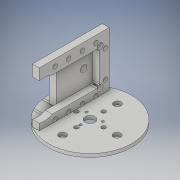
# Autodesk Inventor part: база захвата
Saved by Autodesk Inventor 2019 (Build 230136000, 136)
## iProperties
Created: 2019-08-15
Part Number: база захвата
Material: Типовые
Document SubType Name: Modeling
Designer: Петров Иван
Density: 1 g/cm^3
Appearance: По умолчанию
Author: Петров Иван
Autodesk Inventor part; units mm, degrees
ref_plane "YZ Plane" through (0, 0, 0) normal (1, 0, 0) x (0, 1, 0)
ref_plane "XZ Plane" through (0, 0, 0) normal (0, 1, 0) x (-1, 0, 0)
ref_plane "XY Plane" through (0, 0, 0) normal (0, 0, 1) x (1, 0, 0)
sketch "Эскиз1" plane through (0, 0, 0) normal (0, 1, 0) x (-1, 0, 0)
  circle A0 centre (15.9998, -0.0856) radius 2.1
  circle A1 centre (-15.9998, 0.0856) radius 2.1
  circle A2 centre (0.0856, 15.9998) radius 2.1
  circle A3 centre (-0.0856, -15.9998) radius 2.1
  circle A4 centre (0, 0) radius 2.9
  circle A5 centre (8, 0) radius 1.25
  circle A6 centre (0, 8) radius 1.25
  circle A7 centre (-8, 0) radius 1.25
  circle A8 centre (4.7631, -2.75) radius 0.75
  circle A9 centre (-4.7631, -2.75) radius 0.75
  circle A10 centre (0, 5.5) radius 0.75
  circle A11 centre (0, -8) radius 1.25
  circle A12 centre (0, 0) radius 24.5
  constraints: 13 centre point
extrude "Выдавливание1" add sketch "Эскиз1" along normal blind 2
sketch "Эскиз2" plane through (0, 2, 0) normal (0, 1, 0) x (1, 0, 0)
  line L0 (-13.1408, -20.6607) -> (-9.1408, -20.6607)
  line L1 (-9.1408, -20.6607) -> (-9.1408, 20.3393)
  line L2 (-9.1408, 20.3393) -> (-13.1408, 20.3393)
  line L3 (-13.1408, 20.3393) -> (-13.1408, -20.6607)
  circle A0 centre (0, 0) radius 24.5 projected
  dimension "d2" = 4
  dimension "d3" = 41
  dimension "d4" = 20.3393
  constraints: 8 end point, 2 parallel, 1 horizontal, 1 perpendicular
  measures "d2" distance of L2.end L1.end
  measures "d3" distance of L1.end L0.end
  measures "d4" distance from line of A0.centre L2
extrude "Выдавливание2" add sketch "Эскиз2" along normal blind 32 contours L3 L2 L1 L0
sketch "Эскиз3" plane through (-9.1408, 2, 20.6607) normal (1, 0, 0) x (0, 0, -1)
  line L0 (20.5612, 2.0176) -> (20.5612, -0.2824)
  line L1 (20.5612, 2.0176) -> (21.9612, 2.0176)
  line L2 (21.9612, -0.2824) -> (21.9612, 2.0176)
  line L3 (28.5612, -0.2824) -> (21.9612, -0.2824)
  line L4 (28.5612, 2.0176) -> (28.5612, -0.2824)
  circle A0 centre (2.7612, 14.6176) radius 9.15
  circle A1 centre (2.7612, 14.6176) radius 1.5
  circle A2 centre (38.7612, 22.6176) radius 1.3
  circle A3 centre (25.2612, 28.1176) radius 1.3
  circle A4 centre (33.2612, 28.1176) radius 1.3
  circle A5 centre (17.2612, 28.1176) radius 1.3
  circle A6 centre (9.2612, 28.1176) radius 1.3
  circle A7 centre (38.7612, 6.6176) radius 1.3
  circle A8 centre (25.2612, 1.1176) radius 1.3
  circle A9 centre (33.2612, 1.1176) radius 1.3
  circle A10 centre (17.2612, 1.1176) radius 1.3
  circle A11 centre (9.2612, 1.1176) radius 1.3
  line L5 (-8.2587, 14.5176) -> (-7.7184, 14.5176)
  line L6 (-8.2587, 7.6176) -> (-8.2587, 14.5176)
  arc A12 (-8.2587, 7.6176) -> (-8.2075, 6.8676) centre (-2.7388, 7.6176) ccw
  line L7 (-5.7388, 6.8676) -> (-8.2075, 6.8676)
  arc A13 (-3.9888, 5.1176) -> (-5.7388, 6.8676) centre (-5.7388, 5.1176) ccw
  line L8 (-3.9888, 4.6176) -> (-3.9888, 5.1176)
  line L9 (33.5674, 4.6176) -> (-3.9888, 4.6176)
  arc A14 (33.5674, 4.6176) -> (34.2556, 5.0098) centre (33.5674, 5.4176) ccw
  arc A15 (34.2556, 5.0098) -> (34.869, 5.6231) centre (35.7612, 4.1176) ccw
  arc A16 (34.869, 5.6231) -> (35.2612, 6.3114) centre (34.4612, 6.3114) ccw
  line L10 (35.2612, 22.9239) -> (35.2612, 6.3114)
  arc A17 (35.2612, 22.9239) -> (34.869, 23.6121) centre (34.4612, 22.9239) ccw
  arc A18 (34.2556, 24.2255) -> (34.869, 23.6121) centre (35.7612, 25.1176) ccw
  arc A19 (34.869, 23.6121) -> (34.2556, 24.2255) centre (35.7612, 25.1176) ccw
  line L11 (-3.9888, 3.2947) -> (-3.9888, 4.6176)
  arc A20 (-3.9888, 3.2947) -> (-2.7388, 3.1176) centre (-2.7377, 7.6254) ccw
  line L12 (-2.7388, 3.1176) -> (4.7612, 3.1176)
  line L13 (4.7612, 2.0176) -> (4.7612, 3.1176)
  line L14 (5.9612, 2.0176) -> (4.7612, 2.0176)
  line L15 (5.9612, -0.2824) -> (5.9612, 2.0176)
  line L16 (12.5612, -0.2824) -> (5.9612, -0.2824)
  line L17 (12.5612, 2.0176) -> (12.5612, -0.2824)
  line L18 (13.9612, 2.0176) -> (12.5612, 2.0176)
  line L19 (13.9612, -0.2824) -> (13.9612, 2.0176)
  line L20 (20.5612, -0.2824) -> (13.9612, -0.2824)
  line L21 (20.5612, 2.0176) -> (20.5612, -0.2824)
  line L22 (21.9612, 2.0176) -> (20.5612, 2.0176)
  line L23 (21.9612, -0.2824) -> (21.9612, 2.0176)
  line L24 (28.5612, -0.2824) -> (21.9612, -0.2824)
  line L25 (28.5612, 2.0176) -> (28.5612, -0.2824)
  line L26 (29.9612, 2.0176) -> (28.5612, 2.0176)
  line L27 (29.9612, -0.2824) -> (29.9612, 2.0176)
  line L28 (36.5612, -0.2824) -> (29.9612, -0.2824)
  line L29 (36.5612, 2.0176) -> (36.5612, -0.2824)
  line L30 (37.781, 2.0176) -> (36.5612, 2.0176)
  arc A21 (37.781, 2.0176) -> (37.8612, 2.0978) centre (36.7612, 3.1176) ccw
  line L31 (37.8612, 3.3176) -> (37.8612, 2.0978)
  line L32 (40.1612, 3.3176) -> (37.8612, 3.3176)
  line L33 (40.1612, 9.9176) -> (40.1612, 3.3176)
  line L34 (37.8612, 9.9176) -> (40.1612, 9.9176)
  line L35 (37.8612, 19.3176) -> (37.8612, 9.9176)
  line L36 (40.1612, 19.3176) -> (37.8612, 19.3176)
  line L37 (40.1612, 25.9176) -> (40.1612, 19.3176)
  line L38 (37.8612, 25.9176) -> (40.1612, 25.9176)
  line L39 (37.8612, 27.1374) -> (37.8612, 25.9176)
  arc A22 (37.8612, 27.1374) -> (37.781, 27.2176) centre (36.7612, 26.1176) ccw
  line L40 (36.5612, 27.2176) -> (37.781, 27.2176)
  line L41 (36.5612, 29.5176) -> (36.5612, 27.2176)
  line L42 (29.9612, 29.5176) -> (36.5612, 29.5176)
  line L43 (29.9612, 27.2176) -> (29.9612, 29.5176)
  line L44 (28.5612, 27.2176) -> (29.9612, 27.2176)
  line L45 (28.5612, 29.5176) -> (28.5612, 27.2176)
  line L46 (21.9612, 29.5176) -> (28.5612, 29.5176)
  line L47 (21.9612, 27.2176) -> (21.9612, 29.5176)
  line L48 (20.5612, 27.2176) -> (21.9612, 27.2176)
  line L49 (20.5612, 29.5176) -> (20.5612, 27.2176)
  line L50 (13.9612, 29.5176) -> (20.5612, 29.5176)
  line L51 (13.9612, 27.2176) -> (13.9612, 29.5176)
  line L52 (12.5612, 27.2176) -> (13.9612, 27.2176)
  line L53 (12.5612, 29.5176) -> (12.5612, 27.2176)
  line L54 (5.9612, 29.5176) -> (12.5612, 29.5176)
  line L55 (5.9612, 27.2176) -> (5.9612, 29.5176)
  line L56 (4.7612, 27.2176) -> (5.9612, 27.2176)
  line L57 (4.7612, 26.1176) -> (4.7612, 27.2176)
  line L58 (-2.7388, 26.1176) -> (4.7612, 26.1176)
  arc A23 (-2.7388, 26.1176) -> (-3.9888, 25.9405) centre (-2.7377, 21.6098) ccw
  line L59 (-3.9888, 24.6176) -> (-3.9888, 25.9405)
  line L60 (-3.9888, 24.1176) -> (-3.9888, 24.6176)
  arc A24 (-5.7388, 22.3676) -> (-3.9888, 24.1176) centre (-5.7388, 24.1176) ccw
  line L61 (-8.2075, 22.3676) -> (-5.7388, 22.3676)
  arc A25 (-8.2075, 22.3676) -> (-8.2587, 21.6176) centre (-2.7388, 21.6176) ccw
  line L62 (-8.2587, 14.7176) -> (-8.2587, 21.6176)
  line L63 (-7.7184, 14.7176) -> (-8.2587, 14.7176)
  arc A26 (34.869, 5.6231) -> (34.2556, 5.0098) centre (35.7612, 4.1176) ccw
  arc A27 (34.2556, 24.2255) -> (33.5674, 24.6176) centre (33.5674, 23.8176) ccw
  line L64 (-3.9888, 24.6176) -> (33.5674, 24.6176)
  line L65 (2.7612, 24.6176) -> (2.7612, 23.7676)
  line L66 (2.7612, 5.4676) -> (2.7612, 4.6176)
  point P0 (20.6607, -2)
  point P1 (2.7612, 14.6176)
  constraints: 134 end point, 34 point on circle, 28 centre point, 4 point on line, 1 vertical
extrude "Выдавливание3" cut sketch "Эскиз3" against normal blind 32 contours L66 A0 L65 L64 A27 A18 A17 L10 A16 A26 A14 L9 | A0 | A26 A15 | A19 A18 | A1 | A2 | A3 | A4 | A5 | A6 | A7 | A8 | A9 | A10 | A11
sketch "Эскиз4" plane through (-9.1408, 2, -20.3393) normal (1, 0, 0) x (0, 0, -1)
  arc A0 (-38.2388, 23.7676) -> (-41, 23.3411) centre (-38.2388, 14.6176) ccw projected
  circle A1 centre (-38.2388, 14.6176) radius 11.1
  point P0 (-20.3393, -2)
  dimension "d9" = 22.2
  constraints: 1 centre point, 1 coincident
  measures "d9" diameter of A1
extrude "Выдавливание4" cut sketch "Эскиз4" against normal blind 32
sketch "Эскиз5" plane through (-13.1408, 2, -20.3393) normal (-1, 0, 0) x (0, 0, 1)
  line L0 (3.0085, 26.8076) -> (27.0085, 26.8076)
  line L1 (27.0085, 26.8076) -> (27.0085, 2.8076)
  line L2 (27.0085, 2.8076) -> (3.0085, 2.8076)
  line L3 (3.0085, 2.8076) -> (3.0085, 26.8076)
  point P0 (20.3393, -2)
  dimension "d14" = 24
  dimension "d15" = 24
  constraints: 8 end point, 2 parallel, 1 horizontal, 1 perpendicular
  measures "d14" distance of L0.start L0.end
  measures "d15" distance of L0.end L1.end
extrude "Выдавливание5" add sketch "Эскиз5" along normal blind 4
sketch "Эскиз6" plane through (-17.1408, 2, -20.3393) normal (-1, 0, 0) x (0, 0, 1)
  line L0 (3.0085, 2.8076) -> (27.0085, 2.8076) projected
  line L1 (3.0085, 2.8076) -> (3.0085, 14.6176)
  line L2 (3.0085, 7.6653) -> (3.0085, 21.5699) projected
  line L3 (3.0085, 14.6176) -> (11.0085, 14.6176)
  circle A0 centre (11.0085, 14.6176) radius 2
  point P0 (20.3393, -2)
  dimension "d16" = 8
  dimension "d17" = 4
  constraints: 4 end point, 1 centre point, 1 coincident, 1 midpoint, 1 perpendicular
  measures "d16" distance of L1.end L3.end
  measures "d17" diameter of A0
extrude "Выдавливание6" cut sketch "Эскиз6" against normal blind 5
